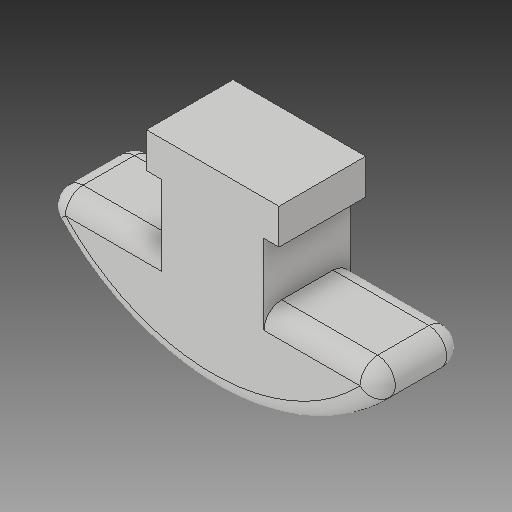
# Autodesk Inventor part: bumper rod
Saved by Autodesk Inventor 2019 (Build 230136000, 136)
## iProperties
Created: 2018-12-04
Part Number: bumper rod
Material: Generic
Document SubType Name: Modeling
Designer: Varga Daniel
Density: 1 g/cm^3
Appearance: Default
Author: Varga Daniel
Autodesk Inventor part; units mm, degrees
ref_plane "YZ Plane" through (0, 0, 0) normal (1, 0, 0) x (0, 1, 0)
ref_plane "XZ Plane" through (0, 0, 0) normal (0, 1, 0) x (-1, 0, 0)
sketch "Sketch1" plane through (0, 0, 0) normal (0, 0, 1) x (1, 0, 0)
  line L0 (-32, -17) -> (17, -17) construction
  line L1 (17, -17) -> (17, -20) construction
  line L2 (29, -20) -> (17, -20) construction
  line L3 (29, -20) -> (29, -17) construction
  line L4 (29, -17) -> (32, -17) construction
  line L5 (32, 17) -> (-32, 17) construction
  line L6 (-32, 17) -> (-32, -17) construction
  circle A0 centre (8, 5) radius 1.65 construction
  circle A1 centre (-14.3, -5.3) radius 1.65 construction
  line L7 (-4.7576, -10.3472) -> (24.4807, -12.9053) construction
  line L8 (24.4807, -12.9053) -> (24.5243, -12.4072) construction
  line L9 (30.5, -17) -> (30.5, -13)
  line L10 (30.5, -13) -> (15.5, -13)
  line L11 (15.5, -13) -> (15.5, -17)
  line L12 (17.2, -17) -> (17.2, -24)
  line L13 (17.2, -24) -> (2.2, -24)
  line L14 (30.5, -17) -> (28.8, -17)
  line L15 (28.8, -17) -> (28.8, -24)
  line L16 (28.8, -24) -> (43.8, -24)
  line L17 (15.5, -17) -> (17.2, -17)
  arc A2 (2.2, -24) -> (43.8, -24) centre (23, -10.1306) ccw
  line L18 (32, -17) -> (32, 17) projected
  point P0 (0, 0)
  dimension "d0" = 0.2
  dimension "d1" = 0.2
  dimension "d2" = 4
  dimension "d3" = 1.7
  dimension "d4" = 1.7
  dimension "d5" = 4
  dimension "d6" = 15
  dimension "d7" = 15
  dimension "d8" = 25
  constraints: 18 end point, 4 perpendicular, 2 collinear, 2 point on circle, 2 point on line, 2 vertical, 1 centre point, 1 horizontal, 1 midpoint
  measures "d0" distance between parallel lines of L12 L1
  measures "d1" distance between parallel lines of L15 L3
  measures "d2" distance between parallel lines of L0 L10
  measures "d3" distance between parallel lines of L15 L9
  measures "d4" distance between parallel lines of L11 L12
  measures "d5" distance between parallel lines of L2 L16
  measures "d6" distance from line of L16.end L15
  measures "d7" distance from line of L13.end L12
  measures "d8" radius of A2
ref_plane "Work Plane1" through (-35, -20, 9.99) normal (0, 0, -1) x (0, 1, 0)
extrude "Extrusion1" add sketch "Sketch1" along normal blind 9.8
fillet "Fillet1" radius 2 8 edges at (23, -35.1306, 0) (2.2, -24, 4.9) (23, -35.1306, 9.8) (43.8, -24, 4.9) (36.3, -24, 0) (9.7, -24, 0) (9.7, -24, 9.8) (36.3, -24, 9.8)
equation "\"d4\" = d3"
equation "\"d7\" = d6"
body "Solid1"
